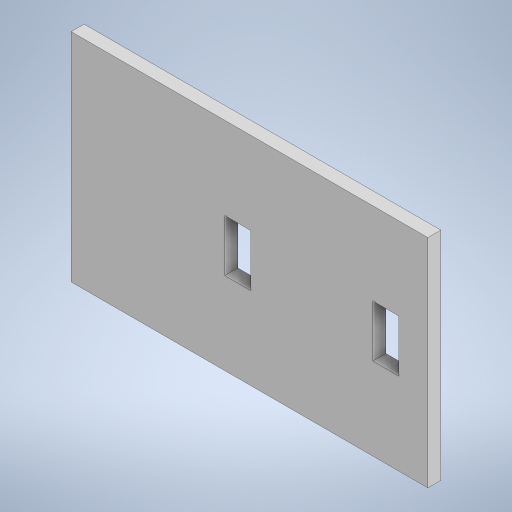
# Autodesk Inventor part: tail plate
Saved by Autodesk Inventor 2024 (Build 280153000, 153)
## iProperties
Created: 2023-07-07
Part Number: tail plate
Material: Generic
Document SubType Name: Modeling
Designer: USER
Density: 1 g/cm^3
Appearance: Default
Author: USER
Autodesk Inventor part; units mm, degrees
ref_plane "YZ Plane" through (0, 0, 0) normal (1, 0, 0) x (0, 1, 0)
ref_plane "XZ Plane" through (0, 0, 0) normal (0, 1, 0) x (-1, 0, 0)
ref_plane "XY Plane" through (0, 0, 0) normal (0, 0, 1) x (1, 0, 0)
sketch "Sketch1" plane through (0, 0, 0) normal (0, 0, 1) x (1, 0, 0)
  line L0 (34.3625, 20.8815) -> (-34.3625, 20.8815)
  line L1 (-34.3625, 20.8815) -> (-34.3625, -20.8815)
  line L2 (-34.3625, -20.8815) -> (34.3625, -20.8815)
  line L3 (34.3625, -20.8815) -> (34.3625, 20.8815)
  point P0 (0, 0)
  constraints: 8 end point, 2 parallel, 1 horizontal, 1 perpendicular
extrude "Extrusion1" add sketch "Sketch1" along normal blind 2.5
sketch "Sketch2" plane through (0, 0, 2.5) normal (0, 0, 1) x (1, 0, 0)
  line L0 (0.2675, 5) -> (-4.7325, 5)
  line L1 (-4.7325, 5) -> (-4.7325, -5)
  line L2 (-4.7325, -5) -> (0.2675, -5)
  line L3 (0.2675, -5) -> (0.2675, 5)
  line L4 (28.7855, 5) -> (23.7855, 5)
  line L5 (23.7855, 5) -> (23.7855, -5)
  line L6 (23.7855, -5) -> (28.7855, -5)
  line L7 (28.7855, -5) -> (28.7855, 5)
  point P0 (0, 0)
  point P1 (-2.2325, 0)
  point P2 (26.2855, 0)
  constraints: 16 end point, 4 parallel, 2 horizontal, 2 perpendicular
extrude "Extrusion2" cut sketch "Sketch2" against normal blind 2.5
body "Solid1"
